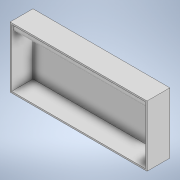
# Autodesk Inventor part: 상자구상도
Saved by Autodesk Inventor 2022.1 (Build 261234000, 234)
## iProperties
Created: 2021-09-06
Part Number: 상자구상도
Material: 일반
Document SubType Name: Modeling
Designer: jwchu
Density: 1 g/cm^3
Appearance: 기본값
Author: jwchu
Autodesk Inventor part; units mm, degrees
ref_plane "YZ Plane" through (0, 0, 0) normal (1, 0, 0) x (0, 1, 0)
ref_plane "XZ Plane" through (0, 0, 0) normal (0, 1, 0) x (-1, 0, 0)
ref_plane "XY Plane" through (0, 0, 0) normal (0, 0, 1) x (1, 0, 0)
sketch "스케치1" plane through (0, 0, 0) normal (0, 0, 1) x (1, 0, 0)
  line L0 (0, 0) -> (900, 0)
  line L1 (900, 0) -> (900, 400)
  line L2 (900, 400) -> (0, 400)
  line L3 (0, 400) -> (0, 0)
  dimension "d2" = 900
  dimension "d3" = 400
  constraints: 8 end point, 2 parallel, 1 horizontal, 1 perpendicular
  measures "d2" distance of L2.end L1.end
  measures "d3" distance of L1.end L0.end
extrude "돌출1" add sketch "스케치1" along normal mid plane 150
sketch "스케치2" plane through (0, 0, 75) normal (0, 0, 1) x (1, 0, 0)
  line L0 (10, 10) -> (890, 10)
  line L1 (890, 10) -> (890, 390)
  line L2 (890, 390) -> (10, 390)
  line L3 (10, 390) -> (10, 10)
  line L4 (0, 400) -> (0, 0) projected
  line L5 (900, 400) -> (0, 400) projected
  line L6 (900, 0) -> (900, 400) projected
  line L7 (900, 0) -> (0, 0) projected
  point P0 (0, 200)
  point P1 (10, 200)
  dimension "d6" = 10
  dimension "d7" = 10
  dimension "d8" = 10
  dimension "d10" = 10
  constraints: 8 end point, 2 midpoint, 2 parallel, 1 horizontal, 1 perpendicular
  measures "d6" distance of point (0, 200) point (10, 200)
  measures "d7" distance between parallel lines of L5 L2
  measures "d8" distance between parallel lines of L6 L1
  measures "d10" distance between parallel lines of L7 L0
extrude "돌출2" cut sketch "스케치2" against normal blind 140 contours L3 L2 L1 L0
sketch "스케치3" plane through (10, 10, 75) normal (1, 0, 0) x (0, 0, -1)
  circle A0 centre (20, 350) radius 11
  line L0 (150, 390) -> (0, 390) projected
  line L1 (0, 390) -> (0, -10) projected
  point P0 (75, -10)
  dimension "d13" = 40
  dimension "d14" = 20
  dimension "d15" = 22
  constraints: 1 centre point
  measures "d13" distance from line of L0 A0.centre
  measures "d14" distance from line of A0.centre L1
  measures "d15" diameter of A0
extrude "돌출3" add sketch "스케치3" along normal blind 880
